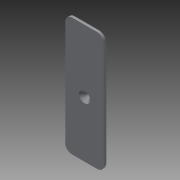
# Autodesk Inventor part: NodeMCU_MQ-7_bottom_shelled
Saved by Autodesk Inventor 2014 SP1 (Build 180222100, 222)
## iProperties
Created: 2016-10-29
Part Number: NodeMCU_MQ-7_bottom_shelled
Material: Generic
Document SubType Name: Modeling
Designer: danielsikar
Density: 1 g/cm^3
Appearance: Default
Author: danielsikar
Autodesk Inventor part; units mm, degrees
ref_plane "YZ Plane" through (0, 0, 0) normal (1, 0, 0) x (0, 1, 0)
ref_plane "XZ Plane" through (0, 0, 0) normal (0, 1, 0) x (-1, 0, 0)
ref_plane "XY Plane" through (0, 0, 0) normal (0, 0, 1) x (1, 0, 0)
sketch "Sketch1" plane through (0, 0, 0) normal (0, 0, 1) x (1, 0, 0)
  line L0 (-16.5, -40.4885) -> (-16.5, 45.3115) projected
  arc A0 (-10, 51.8115) -> (-16.5, 45.3115) centre (-10, 45.3115) ccw projected
  line L1 (-10, 51.8115) -> (10, 51.8115) projected
  arc A1 (16.5, 45.3115) -> (10, 51.8115) centre (10, 45.3115) ccw projected
  line L2 (16.5, 45.3115) -> (16.5, -40.4885) projected
  arc A2 (10.5, -46.4885) -> (16.5, -40.4885) centre (10.5, -40.4885) ccw projected
  line L3 (10.5, -46.4885) -> (-10.5, -46.4885) projected
  arc A3 (-16.5, -40.4885) -> (-10.5, -46.4885) centre (-10.5, -40.4885) ccw projected
  circle A4 centre (0, 0) radius 1.5
  line L4 (-15.8, 45.3115) -> (-15.8, -40.4885)
  arc A5 (-15.8, -40.4885) -> (-10.5, -45.7885) centre (-10.5, -40.4885) ccw
  line L5 (-10.5, -45.7885) -> (10.5, -45.7885)
  arc A6 (10.5, -45.7885) -> (15.8, -40.4885) centre (10.5, -40.4885) ccw
  line L6 (15.8, -40.4885) -> (15.8, 45.3115)
  arc A7 (15.8, 45.3115) -> (10, 51.1115) centre (10, 45.3115) ccw
  line L7 (10, 51.1115) -> (-10, 51.1115)
  arc A8 (-10, 51.1115) -> (-15.8, 45.3115) centre (-10, 45.3115) ccw
  dimension "d0" = 3
  dimension "d1" = 0.7
  constraints: 8 end point, 8 point on circle, 5 centre point, 1 coincident, 7 other
  measures "d0" diameter of A4
  measures "d1" distance between parallel lines of L4 L0
extrude "Extrusion1" add sketch "Sketch1" against normal blind 2 contours A8 L7 A7 L6 A6 L5 A5 L4
sketch "Sketch2" plane through (0, 0, -2) normal (0, 0, -1) x (-1, 0, 0)
  circle A0 centre (0, 0) radius 1.5 projected
  circle A1 centre (0, 0) radius 2.5
  circle A2 centre (0, 0) radius 1.5
  dimension "d4" = 5
  dimension "d5" = 3
  constraints: 2 centre point, 2 coincident
  measures "d4" diameter of A1
  measures "d5" diameter of A2
extrude "Extrusion2" add sketch "Sketch2" along normal blind 9
chamfer "Chamfer1" distance 3 angle 45 1 edges at (-1.5, 0, 0)
body "Solid1"
